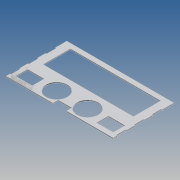
# Autodesk Inventor part: Carosserie_Capot_Avant_Bas
Saved by Autodesk Inventor 2019 (Build 230136000, 136)
## iProperties
Created: 2019-08-27
Part Number: Carosserie_Capot_Avant_Bas
Material: PVC-U
Document SubType Name: Modeling
Designer: jeremias.salamin
Density: 1.4 g/cm^3
Appearance: Lisse - Blanc
Description: Carosserie_Capot_Avant_Bas
Author: jeremias.salamin
Autodesk Inventor part; units mm, degrees
ref_plane "YZ Plane" through (0, 0, 0) normal (1, 0, 0) x (0, 1, 0)
ref_plane "XZ Plane" through (0, 0, 0) normal (0, 1, 0) x (-1, 0, 0)
ref_plane "XY Plane" through (0, 0, 0) normal (0, 0, 1) x (1, 0, 0)
sketch "Sketch1" plane through (0, 0, 0) normal (0, 0, 1) x (1, 0, 0)
  line L0 (0, 35.7) -> (0, -35.7) construction
  line L1 (-63, 0) -> (63, 0) construction
  line L2 (45, -25.5) -> (-45, -25.5)
  line L3 (-45, -25.5) -> (-45, 25.5)
  line L4 (-45, 25.5) -> (45, 25.5)
  line L5 (45, 25.5) -> (45, -25.5)
  line L6 (45, -25.5) -> (-45, 25.5) construction
  line L7 (-45, -25.5) -> (45, 25.5) construction
  point P0 (0, 0)
  dimension "d0" = 90
  dimension "d1" = 51
  constraints: 12 end point, 2 midpoint, 2 parallel, 1 horizontal, 1 perpendicular
  measures "d0" distance of L3.end L4.end
  measures "d1" distance of L2.end L3.end
extrude "Extrusion1" add sketch "Sketch1" along normal mid plane 0.8
sketch "Esquisse2" plane through (0, 0, 0.4) normal (0, 0, 1) x (1, 0, 0)
  line L0 (-45, -25.5) -> (45, -25.5) construction
  line L1 (45, -25.5) -> (45, 25.5) construction
  line L2 (45, 25.5) -> (-45, 25.5) construction
  line L3 (-45, 25.5) -> (-45, -25.5) construction
  line L4 (-63, 0) -> (63, 0) construction
  line L5 (0, 35.7) -> (0, -35.7) construction
  circle A0 centre (-13, -15) radius 9
  circle A1 centre (13, -15) radius 9
  point P0 (0, 0)
  dimension "d4" = 10.5
  dimension "d5" = 18
  dimension "d6" = 18
  dimension "d7" = 26
  constraints: 2 centre point, 1 symmetric about line
  measures "d4" distance from line of L0 A0.centre
  measures "d5" diameter of A0
  measures "d6" diameter of A1
  measures "d7" distance of A1.centre A0.centre
extrude "Extrusion2" cut sketch "Esquisse2" against normal through all
sketch "Esquisse3" plane through (0, 0, 0.4) normal (0, 0, 1) x (1, 0, 0)
  circle A0 centre (-13, -15) radius 9 construction
  circle A1 centre (13, -15) radius 9 construction
  line L0 (-45, -25.5) -> (45, -25.5) construction
  line L1 (45, -25.5) -> (45, 25.5) construction
  line L2 (45, 25.5) -> (-45, 25.5) construction
  line L3 (-45, 25.5) -> (-45, -25.5) construction
  line L4 (-63, 0) -> (63, 0) construction
  line L5 (0, 35.7) -> (0, -35.7) construction
  line L6 (-5.75, -21) -> (5.75, -21)
  line L7 (5.75, -21) -> (5.75, -25.5)
  line L8 (5.75, -25.5) -> (-5.75, -25.5)
  line L9 (-5.75, -25.5) -> (-5.75, -21)
  point P0 (0, 0)
  dimension "d10" = 4.5
  dimension "d11" = 11.5
  constraints: 8 end point, 2 parallel, 1 horizontal, 1 perpendicular, 1 point on line, 1 other
  measures "d10" distance between parallel lines of L0 L6
  measures "d11" distance between parallel lines of L9 L7
extrude "Extrusion3" cut sketch "Esquisse3" against normal through all
sketch "Esquisse4" plane through (0, 0, 0.4) normal (0, 0, 1) x (1, 0, 0)
  line L0 (5.75, -21) -> (5.75, -25.5) construction
  line L1 (5.75, -25.5) -> (45, -25.5) construction
  line L2 (45, -25.5) -> (45, 25.5) construction
  line L3 (45, 25.5) -> (-45, 25.5) construction
  line L4 (-45, 25.5) -> (-45, -25.5) construction
  line L5 (-45, -25.5) -> (-5.75, -25.5) construction
  line L6 (-5.75, -25.5) -> (-5.75, -21) construction
  line L7 (-5.75, -21) -> (5.75, -21) construction
  circle A0 centre (-13, -15) radius 9 construction
  circle A1 centre (13, -15) radius 9 construction
  line L8 (0, 35.7) -> (0, -35.7) construction
  line L9 (-63, 0) -> (63, 0) construction
  line L10 (-38, 21.5) -> (38, 21.5)
  line L11 (38, 21.5) -> (38, -1.5)
  line L12 (38, -1.5) -> (-38, -1.5)
  line L13 (-38, -1.5) -> (-38, 21.5)
  point P0 (0, 0)
  dimension "d14" = 76
  dimension "d15" = 23
  dimension "d16" = 4
  constraints: 8 end point, 2 parallel, 1 horizontal, 1 perpendicular, 1 other
  measures "d14" distance of L11.end L12.end
  measures "d15" distance of L10.end L11.end
  measures "d16" distance between parallel lines of L3 L10
extrude "Extrusion4" cut sketch "Esquisse4" against normal blind 10
sketch "Esquisse5" plane through (0, 0, 0.4) normal (0, 0, 1) x (1, 0, 0)
  line L0 (-38, -1.5) -> (-38, 21.5) construction
  line L1 (-38, 21.5) -> (38, 21.5) construction
  line L2 (38, 21.5) -> (38, -1.5) construction
  line L3 (38, -1.5) -> (-38, -1.5) construction
  line L4 (5.75, -21) -> (5.75, -25.5) construction
  line L5 (5.75, -25.5) -> (45, -25.5) construction
  line L6 (45, -25.5) -> (45, 25.5) construction
  line L7 (45, 25.5) -> (-45, 25.5) construction
  line L8 (-45, 25.5) -> (-45, -25.5) construction
  line L9 (-45, -25.5) -> (-5.75, -25.5) construction
  line L10 (-5.75, -25.5) -> (-5.75, -21) construction
  line L11 (-5.75, -21) -> (5.75, -21) construction
  circle A0 centre (-13, -15) radius 9 construction
  circle A1 centre (13, -15) radius 9 construction
  line L12 (-41, -11.5) -> (-27, -11.5)
  line L13 (-27, -11.5) -> (-27, -21.5)
  line L14 (-27, -21.5) -> (-41, -21.5)
  line L15 (-41, -21.5) -> (-41, -11.5)
  line L16 (0, 35.7) -> (0, -35.7) construction
  line L17 (41, -11.5) -> (27, -11.5)
  line L18 (27, -11.5) -> (27, -21.5)
  line L19 (27, -21.5) -> (41, -21.5)
  line L20 (41, -21.5) -> (41, -11.5)
  point P0 (0, 0)
  dimension "d19" = 14
  dimension "d20" = 10
  dimension "d21" = 4
  dimension "d22" = 4
  constraints: 16 end point, 4 symmetric about line, 2 parallel, 1 horizontal, 1 perpendicular
  measures "d19" distance of L13.end L14.end
  measures "d20" distance of L12.end L13.end
  measures "d21" distance between parallel lines of L9 L14
  measures "d22" distance between parallel lines of L8 L15
extrude "Extrusion5" cut sketch "Esquisse5" against normal blind 10
sketch "Esquisse7" plane through (0, 0, -0.4) normal (0, 0, -1) x (-1, 0, 0)
  line L0 (44.2, 0.8021) -> (45, 0.8021)
  line L1 (45, 0.8021) -> (45, -7.1979)
  line L2 (45, -7.1979) -> (44.2, -7.1979)
  line L3 (44.2, -7.1979) -> (44.2, 0.8021)
  line L4 (44.2, 15.8021) -> (45, 15.8021)
  line L5 (45, 15.8021) -> (45, 7.8021)
  line L6 (45, 7.8021) -> (44.2, 7.8021)
  line L7 (44.2, 7.8021) -> (44.2, 15.8021)
  line L8 (44.2, -14.1979) -> (45, -14.1979)
  line L9 (45, -14.1979) -> (45, -22.1979)
  line L10 (45, -22.1979) -> (44.2, -22.1979)
  line L11 (44.2, -22.1979) -> (44.2, -14.1979)
  line L12 (-45, 0.8021) -> (-44.2, 0.8021)
  line L13 (-44.2, 0.8021) -> (-44.2, -7.1979)
  line L14 (-44.2, -7.1979) -> (-45, -7.1979)
  line L15 (-45, -7.1979) -> (-45, 0.8021)
  line L16 (-45, 15.8021) -> (-44.2, 15.8021)
  line L17 (-44.2, 15.8021) -> (-44.2, 7.8021)
  line L18 (-44.2, 7.8021) -> (-45, 7.8021)
  line L19 (-45, 7.8021) -> (-45, 15.8021)
  line L20 (-45, -14.1979) -> (-44.2, -14.1979)
  line L21 (-44.2, -14.1979) -> (-44.2, -22.1979)
  line L22 (-44.2, -22.1979) -> (-45, -22.1979)
  line L23 (-45, -22.1979) -> (-45, -14.1979)
  point P0 (0, 0)
  constraints: 48 end point, 12 horizontal, 12 vertical, 24 other
extrude "Extrusion7" cut sketch "Esquisse7" against normal blind 0.8
